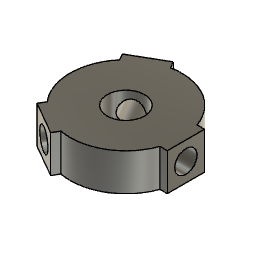
Collar 2 v1 (Autodesk Fusion 360 design; units mm, degrees)
Autodesk Fusion 360 part; units mm, degrees
note: some values were not read from the file. Set by a fixed rule: which sketch regions a step uses.
sketch "Boceto1" plane through (0, 0, 0) normal (0, 0, 1) x (1, 0, 0)
  circle A0 centre (0, 0) radius 2.5
  circle A1 centre (0, 0) radius 7.5
  line L0 (0, 2.5) -> (7.0711, 2.5)
  line L1 (0, -2.5) -> (7.0711, -2.5)
  line L2 (7.0711, 2.5) -> (7.0711, -2.5)
  line L3 (7.0711, 2.5) -> (8.0711, 2.5)
  line L4 (8.0711, 2.5) -> (8.0711, -2.5)
  line L5 (8.0711, -2.5) -> (7.0711, -2.5)
  line L6 (-6.2006, 5.7397) -> (-1.8705, 8.2397)
  line L7 (-5.7006, 4.8737) -> (-6.2006, 5.7397)
  line L8 (-1.8705, 8.2397) -> (-1.3705, 7.3737)
  line L9 (-1.8705, -8.2397) -> (-6.2006, -5.7397)
  line L10 (-1.3705, -7.3737) -> (-1.8705, -8.2397)
  line L11 (-6.2006, -5.7397) -> (-5.7006, -4.8737)
  dimension "d1" = 5
  dimension "d2" = 15
  dimension "d3" = 1
  dimension "d5" = 360
  constraint coincident A0.centre A1.centre
  constraint concentric A0 A1
  constraint coincident A0 L0.start
  constraint coincident A1 L0.end
  constraint horizontal L0
  constraint coincident A0 L1.start
  constraint coincident A1 L1.end
  constraint parallel L0 L1
  constraint perpendicular L1 L2
  constraint perpendicular L2 L3
  constraint perpendicular L3 L4
  constraint perpendicular L2 L5
  measures "d1" diameter of A0
  measures "d2" diameter of A1
  measures "d3" distance of L0.end L3.end
extrude "Extruir1" add sketch "Boceto1" along normal blind 5 contours A0 L0 L1 L2 | A0 A1 L0 L1 | A1 L3 L4 L5 | A1 L2 | A1 L6 L7 L8 | A1 L9 L10 L11
sketch "Boceto2" plane through (-4.0355, -6.9897, 0) normal (-0.5, -0.866025, 0) x (0.866025, -0.5, 0)
  line L0 (-2.5, 0) -> (2.5, 0)
  line L1 (2.5, 0) -> (2.5, 5)
  line L2 (2.5, 5) -> (-2.5, 5)
  line L3 (-2.5, 5) -> (-2.5, 0)
  line L4 (-2.5, 5) -> (2.5, 0)
  line L5 (2.5, 5) -> (-2.5, 0)
  circle A0 centre (0, 2.5) radius 1.5
  dimension "d8" = 3
  constraint coincident L2.end L3.start
  constraint coincident L0.end L1.start
  constraint coincident L1.end L2.start
  constraint coincident L0.start L3.end
  constraint midpoint L5 A0.centre
  measures "d8" diameter of A0
sketch "Boceto3" plane through (8.0711, 0, 0) normal (1, 0, 0) x (0, 1, 0)
  line L0 (-2.5, 0) -> (2.5, 0)
  line L1 (2.5, 0) -> (2.5, 5)
  line L2 (2.5, 5) -> (-2.5, 5)
  line L3 (-2.5, 5) -> (-2.5, 0)
  line L4 (-2.5, 5) -> (2.5, 0)
  line L5 (2.5, 5) -> (-2.5, 0)
  circle A0 centre (0, 2.5) radius 1.5
  dimension "d9" = 3
  constraint coincident L2.end L3.start
  constraint coincident L0.end L1.start
  constraint coincident L1.end L2.start
  constraint coincident L0.start L3.end
  constraint midpoint L5 A0.centre
  measures "d9" diameter of A0
sketch "Boceto4" plane through (-4.0355, 6.9897, 0) normal (-0.5, 0.866025, 0) x (-0.866025, -0.5, 0)
  line L0 (-2.5, 0) -> (2.5, 0)
  line L1 (2.5, 0) -> (2.5, 5)
  line L2 (2.5, 5) -> (-2.5, 5)
  line L3 (-2.5, 5) -> (-2.5, 0)
  line L4 (2.5, 5) -> (-2.5, 0)
  line L5 (-2.5, 5) -> (2.5, 0)
  circle A0 centre (0, 2.5) radius 1.5
  dimension "d10" = 3
  constraint coincident L1.end L2.start
  constraint coincident L0.start L3.end
  constraint coincident L2.end L3.start
  constraint coincident L0.end L1.start
  constraint midpoint L5 A0.centre
  measures "d10" diameter of A0
extrude "Extruir2" cut sketch "Boceto4" against normal blind 8 contours L4 L5 A0 | L4 L5 A0 | L4 L5 A0 | L4 L5 A0
extrude "Extruir3" cut sketch "Boceto2" against normal blind 8 contours L4 L5 A0 | L4 L5 A0 | L4 L5 A0 | L4 L5 A0
extrude "Extruir4" cut sketch "Boceto3" against normal blind 8 contours L4 L5 A0 | L4 L5 A0 | L4 L5 A0 | L4 L5 A0
